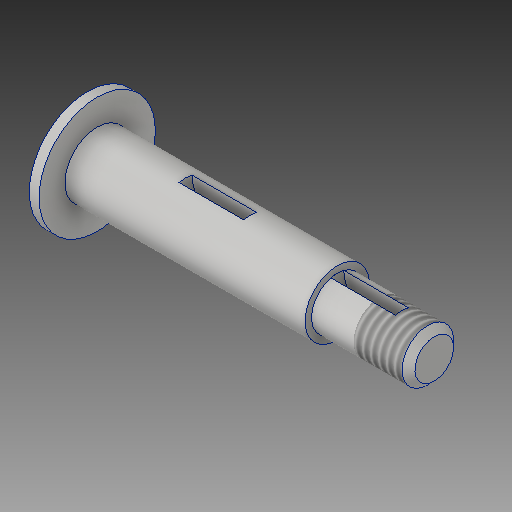
# Autodesk Inventor part: Flecha del engrane
Saved by Autodesk Inventor 2020 (Build 240168000, 168)
## iProperties
Created: 2016-05-04
Part Number: Flecha del engrane
Material: Aluminum 6061
Document SubType Name: Modeling
Designer: Jorge
Density: 2.7 g/cm^3
Appearance: Aluminum - Flat
Mass: 43.8959 g
Surface Area: 57.9757 cm^2
Volume: 16.2578 cm^3
Author: Jorge
Autodesk Inventor part; units mm, degrees
ref_plane "YZ Plane" through (0, 0, 0) normal (1, 0, 0) x (0, 1, 0)
ref_plane "XZ Plane" through (0, 0, 0) normal (0, 1, 0) x (-1, 0, 0)
ref_plane "XY Plane" through (0, 0, 0) normal (0, 0, 1) x (1, 0, 0)
sketch "Sketch1" plane through (0, 0, 0) normal (0, 0, 1) x (1, 0, 0)
  line L0 (58.9915, 7.9216) -> (58.9915, 6.3309)
  line L1 (58.9915, 6.3309) -> (82.804, 6.3309)
  line L2 (-22.9853, 0) -> (100.4355, 0) projected
  line L3 (0, 7.9216) -> (58.9915, 7.9216)
  line L4 (0, 0) -> (0, 14.2875) construction
  line L5 (0, -5.5981) -> (0, 33.5884) construction
  line L6 (0, 14.2875) -> (0, 7.9216)
  line L7 (82.804, 6.3309) -> (82.804, 0)
  line L8 (-4.7625, 0) -> (82.804, 0)
  line L9 (-4.7625, 0) -> (-4.7625, 27.9903) construction
  line L10 (0, 14.2875) -> (-2.3813, 14.2875)
  arc A0 (-2.3813, 14.2875) -> (-4.7625, 0) centre (39.2906, 0) ccw
  dimension "d4" = 15.8432
  dimension "d6" = 23.8125
  dimension "d8" = 58.9915
  dimension "d9" = 12.6619
  dimension "d10" = 0
  dimension "d16" = 2.3813
  dimension "d17" = 2.3813
  dimension "d18" = 28.575
  constraints: 18 end point, 3 horizontal, 3 perpendicular, 3 point on line, 2 point on circle, 1 centre point, 1 collinear, 1 tangent, 1 vertical
  measures "d4" diameter of L3 L2
  measures "d6" distance from line of L1.end L0
  measures "d8" horizontal distance of L0.start L4.end
  measures "d9" diameter of L1 L2
  measures "d10" distance between parallel lines of L4 L5
  measures "d16" distance of L4.end L10.end
  measures "d17" distance from line of L9 L10.end
  measures "d18" diameter of L10 L2
revolve "Revolution1" add sketch "Sketch1" angle 360 about axis through (-10, 0, 0) along (1, 0, 0)
sketch "Sketch2" plane through (0, 0, 0) normal (0, 0, 1) x (1, 0, 0)
  circle A0 centre (29.6227, 7.9216) radius 7.9375
  circle A1 centre (66.929, 6.3309) radius 7.9375
  line L0 (58.9915, -7.9216) -> (58.9915, 7.9216) construction
  line L1 (0, 7.9216) -> (58.9915, 7.9216) construction
  line L2 (58.9915, 6.3309) -> (82.804, 6.3309) construction
  point P0 (0, 0)
  dimension "d20" = 29.3687
  dimension "d21" = 7.9375
  dimension "d22" = 15.875
  dimension "d23" = 0
  dimension "d24" = 0
  constraints: 2 centre point, 1 equal radius
  measures "d20" distance from line of A0.centre L0
  measures "d21" distance from line of A1.centre L0
  measures "d22" diameter of A0
  measures "d23" distance from line of L1 A0.centre
  measures "d24" distance from line of L2 A1.centre
extrude "Extrusion1" cut sketch "Sketch2" along normal mid plane 3.175
chamfer "Chamfer1" distance 1.5875 angle 45 1 edges at (82.804, -6.3309, 0)
thread "Thread1" size "1/2-13 UNC" class "2A" standard "ANSI Unified Screw Threads" length 11.9062
equation "\"d17\" = d16"
body "Solid1"
